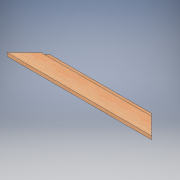
# Autodesk Inventor part: SkirtWidth
Saved by Autodesk Inventor 2016 (Build 200138000, 138)
## iProperties
Created: 2016-02-11
Part Number: SkirtWidth
Material: Wood (Birch)
Document SubType Name: Modeling
Designer: ron
Density: 0.55 g/cm^3
Appearance: Birch - Natural Polished
Mass: 939.194 g
Surface Area: 2236.29 cm^2
Volume: 1707.63 cm^3
Author: ron
Autodesk Inventor part; units mm, degrees
ref_plane "YZ Plane" through (0, 0, 0) normal (1, 0, 0) x (0, 1, 0)
ref_plane "XZ Plane" through (0, 0, 0) normal (0, 1, 0) x (-1, 0, 0)
ref_plane "XY Plane" through (0, 0, 0) normal (0, 0, 1) x (1, 0, 0)
sketch "Sketch1" plane through (0, 0, 0) normal (1, 0, 0) x (0, 1, 0)
  line L0 (0, 0) -> (0, -127)
  line L1 (0, -127) -> (10, -127)
  line L2 (10, -127) -> (10, -101.6)
  line L3 (10, -101.6) -> (20, -101.6)
  line L4 (20, -101.6) -> (20, 0)
  line L5 (20, 0) -> (0, 0)
  dimension "d0" = 127
  dimension "d1" = 10
  dimension "d2" = 25.4
  dimension "d3" = 10
  constraints: 12 end point, 5 perpendicular, 1 vertical
  measures "d0" distance of L0.start L0.end
  measures "d1" distance of L0.end L1.end
  measures "d2" distance of L1.end L2.end
  measures "d3" distance of L2.end L3.end
extrude "Extrusion1" add sketch "Sketch1" along normal blind 863.6
chamfer "Chamfer1" distance 127 angle 45 1 edges at (863.6, 5, -127)
chamfer "Chamfer2" distance 127 angle 45 1 edges at (0, 5, -127)
sketch "Sketch2" plane through (0, 0, 0) normal (0, -1, 0) x (1, 0, 0)
  line L0 (101.6, -101.6) -> (762, -101.6) projected
  line L1 (736.6, -127) -> (762, -101.6)
  line L2 (863.6, 0) -> (736.6, -127) projected
  line L3 (762, -101.6) -> (762, -76.2)
  line L4 (762, -76.2) -> (787.4, -76.2)
  point P0 (0, 0)
  dimension "d12" = 25.4
  dimension "d13" = 25.4
  dimension "d14" = 90
  constraints: 6 end point, 1 collinear, 1 point on line
  measures "d12" distance of L0.end L3.end
  measures "d13" distance of L3.end L4.end
  measures "d14" angle of L3 L4
sketch "Sketch3" plane through (0, 0, 0) normal (0, -1, 0) x (1, 0, 0)
  line L0 (0, 0) -> (101.6, -101.6) projected
  line L1 (101.6, -101.6) -> (101.6, -76.2)
  line L2 (101.6, -76.2) -> (76.2, -76.2)
  dimension "d15" = 25.4
  constraints: 4 end point, 1 perpendicular, 1 point on line, 1 vertical
  measures "d15" distance of L0.end L1.end
extrude "Extrusion2" cut sketch "Sketch2" against normal blind 3.175
extrude "Extrusion3" cut sketch "Sketch3" against normal blind 3.175
body "Solid1"
